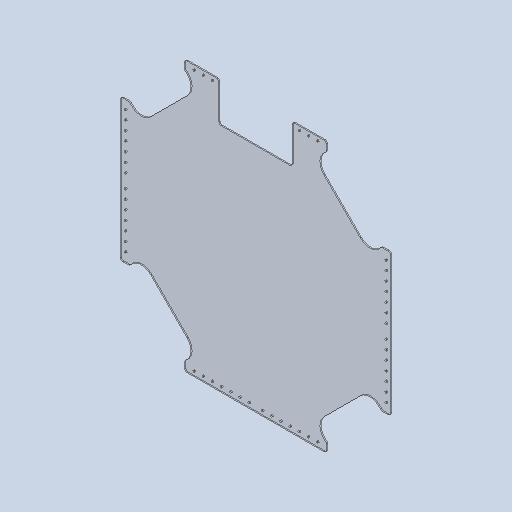
# Autodesk Inventor part: BellyPanBot
Saved by Autodesk Inventor 2025.2 (Build 292293000, 293)
## iProperties
Created: 2025-01-13
Part Number: BellyPanBot
Material: Lexan, Clear
Document SubType Name: Sheet Metal
Designer: Marcus Tannini
Density: 1.2 g/cm^3
Appearance: Lexan (Clear)
Mfg Approved By: John.Thibert
Sheet Metal Rule: Default
Mass: 1686.5 g
Surface Area: 8971.77 cm^2
Volume: 1405.41 cm^3
ILogicPurgeVersion: 0.0.0.0
OnSaveVersion: 3.4.0.0
OnSaveAssembly: COREAutomationManager
ModelCat: Uncategorized
MaterialName: Lexan, Clear
CN_MASS: 1.6
Author: Marcus Tannini
Autodesk Inventor part; units mm, degrees
ref_plane "YZ Plane" through (0, 0, 0) normal (1, 0, 0) x (0, 1, 0)
ref_plane "XZ Plane" through (0, 0, 0) normal (0, 1, 0) x (-1, 0, 0)
ref_plane "XY Plane" through (0, 0, 0) normal (0, 0, 1) x (1, 0, 0)
sketch "Sketch5" plane through (0, 0, 0) normal (0, 0, 1) x (1, 0, 0)
  line L0 (-374.65, 374.65) -> (374.65, 374.65)
  line L1 (374.65, 374.65) -> (374.65, -374.65)
  line L2 (374.65, -374.65) -> (-374.65, -374.65)
  line L3 (-374.65, -374.65) -> (-374.65, 374.65)
  line L4 (-374.65, 374.65) -> (374.65, -374.65) construction
  line L5 (374.65, 374.65) -> (-374.65, -374.65) construction
  line L6 (374.65, 196.85) -> (349.25, 196.85)
  arc A0 (291.385, 189.7435) -> (349.25, 196.85) centre (317.5415, 215.9) ccw
  line L7 (291.385, 189.7435) -> (189.7435, 291.385)
  line L8 (196.85, 374.65) -> (196.85, 349.25)
  arc A1 (196.85, 349.25) -> (189.7435, 291.385) centre (215.9, 317.5415) ccw
  point P0 (0, 0)
  point P1 (240.5642, 240.5642)
  point P2 (196.85, 374.65)
  dimension "d22" = 749.3
  dimension "d23" = 749.3
  dimension "d24" = 177.8
  dimension "d27" = 25.4
  dimension "d29" = 36.9909
  dimension "d31" = 158.75
  constraints: 18 end point, 4 point on circle, 3 midpoint, 3 perpendicular, 3 symmetric about line, 2 centre point, 2 parallel, 2 point on line, 1 horizontal, 1 tangent, 1 other
  measures "d22" distance of L1.end L2.end
  measures "d23" distance of L0.end L1.end
  measures "d24" distance between parallel lines of L0 L6
  measures "d27" distance of L6.start L6.end
  measures "d29" radius of A0
  measures "d31" distance from line of L0 A0.centre
extrude "Plate1" add sketch "Sketch5" along normal mid plane 3.175
extrude "Extrusion3" cut sketch "Sketch5" along normal through all both and the other way through all contours L0 L1 L6 A0 L7 A1 L8
fillet "Corner Round1" radius 6.35 2 edges at (349.25, 196.85, 0) (196.85, 349.25, 0)
pattern_circular "Circular Pattern1" count 4 over 360 about axis through (0, 0, -10) along (0, 0, 1) of "Extrusion3", "Corner Round1"
fillet "Corner Round2" radius 6 8 edges at (374.65, 196.85, 0) (196.85, 374.65, 0) (-196.85, 374.65, 0) (-374.65, 196.85, 0) (-374.65, -196.85, 0) (-196.85, -374.65, 0) (196.85, -374.65, 0) (374.65, -196.85, 0)
sketch "Sketch6" plane through (0, 0, -1.5875) normal (0, 0, -1) x (-1, 0, 0)
  line L0 (-352.6596, 196.85) -> (-368.65, 196.85) construction
  line L1 (-374.65, -190.85) -> (-374.65, 190.85) construction
  point P0 (0, 0)
  point P1 (-361.95, 19.05)
  dimension "d40" = 177.8
  dimension "d41" = 12.7
  measures "d40" distance from line of L0 point (-361.95, 19.05)
  measures "d41" distance from line of point (-361.95, 19.05) L1
hole "Hole1" at (361.95, 19.05, -1.5875) direction (0, 0, 1) diameter 4.9784 end through all clearance for "Flat Head Machine Screw (82)" size "#10" standard "Ansi Unified Screw Threads"
pattern_linear "Rectangular Pattern1" count 7 spacing 25.4 along (0, 1, 0) of "Hole1"
mirror "Mirror1" about plane through (0, 0, 0) normal (0, 1, 0) of "Hole1", "Rectangular Pattern1"
pattern_circular "Circular Pattern2" count 4 over 360 about axis through (0, 0, -10) along (0, 0, 1) of "Hole1", "Rectangular Pattern1", "Mirror1"
sketch "Sketch7" plane through (0, 0, -1.5875) normal (0, 0, -1) x (-1, 0, 0)
  line L0 (101.6, 374.65) -> (-101.6, 374.65)
  line L1 (-101.6, 374.65) -> (-101.6, 266.7)
  line L2 (-101.6, 266.7) -> (101.6, 266.7)
  line L3 (101.6, 266.7) -> (101.6, 374.65)
  line L4 (101.6, 374.65) -> (-101.6, 266.7) construction
  line L5 (-101.6, 374.65) -> (101.6, 266.7) construction
  line L6 (-190.85, 374.65) -> (190.85, 374.65) construction
  line L7 (-524.51, 0) -> (524.51, 0) construction
  line L8 (0, -524.51) -> (0, 524.51) construction
  point P0 (0, 0)
  point P1 (0, 320.675)
  dimension "d55" = 107.95
  dimension "d56" = 203.2
  constraints: 12 end point, 2 midpoint, 2 parallel, 1 collinear, 1 horizontal, 1 perpendicular, 1 point on line
  measures "d55" distance of L2.end L0.start
  measures "d56" distance of L1.end L2.end
extrude "Cut1" cut sketch "Sketch7" against normal blind 3.175
fillet "Corner Round3" radius 6.35 4 edges at (-101.6, 374.65, 0) (101.6, 374.65, 0) (-101.6, 266.7, 0) (101.6, 266.7, 0)
equation "\"d47\" = Thickness"
equation "\"d57\" = Thickness"
equation "\"d32\" = Thickness"
equation "\"BendRadius\" = Thickness"
equation "\"BendReliefWidth\" = Thickness"
equation "\"BendReliefDepth\" = 0.5 * Thickness"
equation "\"CornerReliefSize\" = 4 * Thickness"
equation "\"MinimumRemnant\" = 2 * Thickness"
equation "\"TransitionRadius\" = BendRadius"
equation "\"JacobiRadiusSize\" = BendRadius"
equation "\"GapSize\" = Thickness"
equation "\"Thickness\" = 3.175"
body "Solid2"
